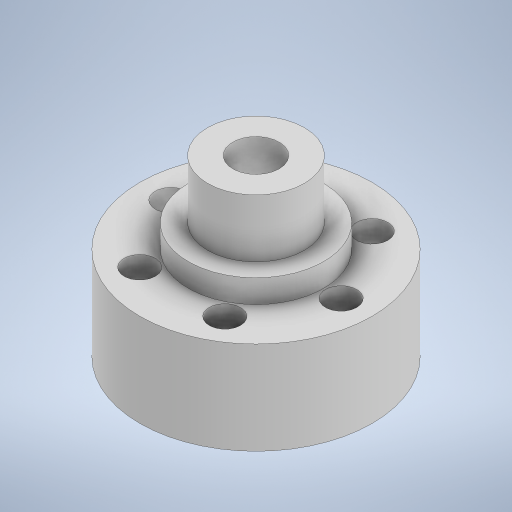
# Autodesk Inventor part: MiniPodsipnikNatag
Saved by Autodesk Inventor 2024 (Build 280153000, 153)
## iProperties
Created: 2023-08-26
Part Number: MiniPodsipnikNatag
Material: Generic
Document SubType Name: Modeling
Designer: KirikDK
Density: 1 g/cm^3
Appearance: Default
Author: KirikDK
Autodesk Inventor part; units mm, degrees
ref_plane "YZ Plane" through (0, 0, 0) normal (1, 0, 0) x (0, 1, 0)
ref_plane "XZ Plane" through (0, 0, 0) normal (0, 1, 0) x (-1, 0, 0)
ref_plane "XY Plane" through (0, 0, 0) normal (0, 0, 1) x (1, 0, 0)
sketch "Sketch1" plane through (0, 0, 0) normal (0, 1, 0) x (-1, 0, 0)
  circle A0 centre (0, 0) radius 17.5
  dimension "d0" = 35
  constraints: 1 centre point, 1 coincident
  measures "d0" diameter of A0
extrude "Extrusion1" add sketch "Sketch1" along normal blind 6
sketch "Sketch2" plane through (0, 6, 0) normal (0, 1, 0) x (1, 0, 0)
  circle A0 centre (0, 0) radius 12.5
  dimension "d3" = 25
  constraints: 1 centre point, 1 coincident
  measures "d3" diameter of A0
extrude "Extrusion2" add sketch "Sketch2" along normal blind 15
sketch "Sketch3" plane through (0, 21, 0) normal (0, 1, 0) x (1, 0, 0)
  circle A0 centre (0, 0) radius 6
  constraints: 1 centre point, 1 coincident
extrude "Extrusion3" cut sketch "Sketch3" against normal blind 100
sketch "Sketch4" plane through (0, 0, 0) normal (0, -1, 0) x (1, 0, 0)
  circle A0 centre (0, 0) radius 6
  circle A1 centre (0, 0) radius 30
  circle A2 centre (22, 0) radius 4.05
  circle A3 centre (11, 19.0526) radius 4.05
  circle A4 centre (-11, 19.0526) radius 4.05
  circle A5 centre (-22, 0) radius 4.05
  circle A6 centre (-11, -19.0526) radius 4.05
  circle A7 centre (11, -19.0526) radius 4.05
  dimension "d8" = 60
  dimension "d11" = 12
  dimension "d12" = 22
  dimension "d13" = 8.1
  dimension "d16" = 360
  constraints: 8 centre point, 2 coincident, 13 other
  measures "d8" diameter of A1
  measures "d11" diameter of A0
  measures "d12" distance of point (0, 0) A2.centre
  measures "d13" diameter of A2
extrude "Extrusion4" add sketch "Sketch4" along normal blind 24
body "Solid1"
